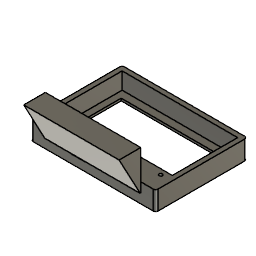
inky_case (Autodesk Fusion 360 design; units mm, degrees)
Autodesk Fusion 360 part; units mm, degrees
sketch "Sketch1" plane through (0, 0, 0) normal (0, 0, 1) x (1, 0, 0)
  line L0 (-52.4, -38.35) -> (52.4, -38.35)
  line L1 (52.4, -38.35) -> (52.4, 38.35)
  line L2 (52.4, 38.35) -> (-52.4, 38.35)
  line L3 (-52.4, 38.35) -> (-52.4, -38.35)
extrude "Extrude1" add sketch "Sketch1" along normal blind 16 makes body 1
ref_plane "WorkPlane1" through (0, 0, 2) normal (0, 0, 1) x (1, 0, 0)
sketch "Sketch2" plane through (0, 0, 2) normal (0, 0, 1) x (1, 0, 0)
  line L0 (-48.4, -34.35) -> (48.4, -34.35)
  line L1 (48.4, -34.35) -> (48.4, 34.35)
  line L2 (48.4, 34.35) -> (-48.4, 34.35)
  line L3 (-48.4, 34.35) -> (-48.4, -34.35)
extrude "Extrude2" add sketch "Sketch2" along normal blind 15 separate body makes body 2
combine "Combine1" operation cut target body 1 tool bodies 2
ref_plane "WorkPlane2" through (0, 0, -1) normal (0, 0, 1) x (1, 0, 0)
sketch "Sketch3" plane through (0, 0, -1) normal (0, 0, 1) x (1, 0, 0)
  line L0 (-43, -25.85) -> (43, -25.85)
  line L1 (43, -25.85) -> (43, 28.15)
  line L2 (43, 28.15) -> (-43, 28.15)
  line L3 (-43, 28.15) -> (-43, -25.85)
extrude "Extrude3" add sketch "Sketch3" along normal blind 4 separate body makes body 3
combine "Combine2" operation cut target body 1 tool bodies 3
ref_plane "WorkPlane3" through (0, 0, 13.5) normal (0, 0, 1) x (1, 0, 0)
sketch "Sketch4" plane through (0, 0, 13.5) normal (0, 0, 1) x (1, 0, 0)
  line L0 (-52.4, -38.35) -> (52.4, -38.35)
  line L1 (52.4, -38.35) -> (52.4, -20.35)
  line L2 (52.4, -20.35) -> (-52.4, -20.35)
  line L3 (-52.4, -20.35) -> (-52.4, -38.35)
extrude "Extrude4" add sketch "Sketch4" along normal blind 2.5 separate body makes body 4
combine "Combine3" operation add target body 1 tool bodies 4
ref_plane "WorkPlane4" through (0, 0, 13) normal (0, 0, 1) x (1, 0, 0)
sketch "Sketch5" plane through (0, 0, 13) normal (0, 0, 1) x (1, 0, 0)
  circle A0 centre (-43.2, -24.85) radius 1.4
extrude "Extrude5" add sketch "Sketch5" along normal blind 3.5 separate body makes body 5
combine "Combine4" operation cut target body 1 tool bodies 5
ref_plane "WorkPlane5" through (0, 0, 13) normal (0, 0, 1) x (1, 0, 0)
sketch "Sketch6" plane through (0, 0, 13) normal (0, 0, 1) x (1, 0, 0)
  circle A0 centre (43.18, -24.85) radius 1.4
extrude "Extrude6" add sketch "Sketch6" along normal blind 3.5 separate body makes body 6
combine "Combine5" operation cut target body 1 tool bodies 6
ref_plane "WorkPlane6" through (0, -38.85, 0) normal (0, 1, 0) x (0, 0, 1)
sketch "Sketch7" plane through (0, -38.85, 0) normal (0, 1, 0) x (1, 0, 0)
  line L0 (-18.7, -7.2) -> (-6.3, -7.2)
  line L1 (-6.3, -7.2) -> (-6.3, -17.8)
  line L2 (-6.3, -17.8) -> (-18.7, -17.8)
  line L3 (-18.7, -17.8) -> (-18.7, -7.2)
extrude "Extrude7" add sketch "Sketch7" along normal blind 5 separate body makes body 7
combine "Combine6" operation cut target body 1 tool bodies 7
ref_plane "WorkPlane7" through (0, -38.85, 0) normal (0, 1, 0) x (0, 0, 1)
sketch "Sketch8" plane through (0, -38.85, 0) normal (0, 1, 0) x (1, 0, 0)
  line L0 (-35, -8) -> (-25, -8)
  line L1 (-25, -8) -> (-25, -11)
  line L2 (-25, -11) -> (-35, -11)
  line L3 (-35, -11) -> (-35, -8)
extrude "Extrude8" add sketch "Sketch8" along normal blind 5 separate body makes body 8
combine "Combine7" operation cut target body 1 tool bodies 8
ref_plane "WorkPlane8" through (0, -38.85, 0) normal (0, 1, 0) x (0, 0, 1)
sketch "Sketch9" plane through (0, -38.85, 0) normal (0, 1, 0) x (1, 0, 0)
  line L0 (25, -8) -> (35, -8)
  line L1 (35, -8) -> (35, -11)
  line L2 (35, -11) -> (25, -11)
  line L3 (25, -11) -> (25, -8)
extrude "Extrude9" add sketch "Sketch9" along normal blind 5 separate body makes body 9
combine "Combine8" operation cut target body 1 tool bodies 9
fillet "Fillet1" radius 2 4 edges at (-52.4, -38.35, 8) (52.4, -38.35, 8) (-52.4, 38.35, 8) (52.4, 38.35, 8) on bodies 1
ref_plane "WorkPlane9" through (-40, 0, 0) normal (1, 0, 0) x (0, 1, 0)
sketch "Sketch10" plane through (-40, 0, 0) normal (1, 0, 0) x (0, 0, -1)
  line L0 (-7, -38.35) -> (-41, -38.35)
  line L1 (-41, -38.35) -> (-41, -56.55)
  line L2 (-41, -56.55) -> (-7, -38.35)
extrude "Extrude10" add sketch "Sketch10" along normal blind 80 separate body makes body 10
ref_plane "WorkPlane10" through (0, -38.35, 0) normal (0, 1, 0) x (0, 0, 1)
sketch "Sketch11" plane through (0, -38.35, 0) normal (0, 1, 0) x (1, 0, 0)
  line L0 (-34.8, -8.15) -> (-25.2, -8.15)
  line L1 (-25.2, -8.15) -> (-25.2, -10.85)
  line L2 (-25.2, -10.85) -> (-34.8, -10.85)
  line L3 (-34.8, -10.85) -> (-34.8, -8.15)
extrude "Extrude11" add sketch "Sketch11" along normal blind 3.6 separate body makes body 11
combine "Combine9" operation add target body 10 tool bodies 11
ref_plane "WorkPlane11" through (0, -38.35, 0) normal (0, 1, 0) x (0, 0, 1)
sketch "Sketch12" plane through (0, -38.35, 0) normal (0, 1, 0) x (1, 0, 0)
  line L0 (25.2, -8.15) -> (34.8, -8.15)
  line L1 (34.8, -8.15) -> (34.8, -10.85)
  line L2 (34.8, -10.85) -> (25.2, -10.85)
  line L3 (25.2, -10.85) -> (25.2, -8.15)
extrude "Extrude12" add sketch "Sketch12" along normal blind 3.6 separate body makes body 12
combine "Combine10" operation add target body 10 tool bodies 12
chamfer "Chamfer1" distance 1 angle 45 1 edges at (0, -38.35, 7) on bodies 10
